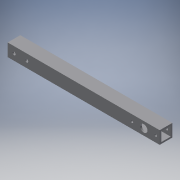
# Autodesk Inventor part: 1x1x12
Saved by Autodesk Inventor 2016 (Build 200138000, 138)
## iProperties
Created: 2016-01-17
Part Number: 1x1x12
Material: Aluminum 6061
Document SubType Name: Modeling
Designer: gus
Density: 2.7 g/cm^3
Appearance: Aluminum - Flat
Mass: 227.61 g
Surface Area: 544.154 cm^2
Volume: 84.2999 cm^3
User Status: complete
Author: gus
Autodesk Inventor part; units mm, degrees
ref_plane "YZ Plane" through (0, 0, 0) normal (1, 0, 0) x (0, 1, 0)
ref_plane "XZ Plane" through (0, 0, 0) normal (0, 1, 0) x (-1, 0, 0)
ref_plane "XY Plane" through (0, 0, 0) normal (0, 0, 1) x (1, 0, 0)
sketch "Sketch1" plane through (0, 0, 0) normal (1, 0, 0) x (0, 1, 0)
  line L0 (0, 0) -> (25.4, 0)
  line L1 (25.4, 0) -> (25.4, -25.4)
  line L2 (25.4, -25.4) -> (0, -25.4)
  line L3 (0, -25.4) -> (0, 0)
  line L4 (22.225, -3.175) -> (3.175, -3.175)
  line L5 (3.175, -3.175) -> (3.175, -22.225)
  line L6 (3.175, -22.225) -> (22.225, -22.225)
  line L7 (22.225, -22.225) -> (22.225, -3.175)
  dimension "d0" = 25.4
  dimension "d1" = 25.4
  dimension "d2" = 3.175
  constraints: 16 end point, 4 parallel, 2 perpendicular, 1 horizontal, 3 other
  measures "d0" distance of L1.end L2.end
  measures "d1" distance of L0.end L1.end
  measures "d2" distance between parallel lines of L0 L4
extrude "Extrusion1" add sketch "Sketch1" along normal blind 304.8
sketch "Sketch2" plane through (0, 0, 0) normal (0, 0, 1) x (1, 0, 0)
  circle A0 centre (273.05, 12.7) radius 23.8125 construction
  line L0 (0, 25.4) -> (304.8, 25.4) construction
  line L1 (304.8, 25.4) -> (304.8, 0) construction
  circle A1 centre (296.8625, 12.7) radius 2.54
  circle A2 centre (249.2375, 12.7) radius 2.54
  line L2 (304.8, 12.7) -> (0, 12.7) construction
  line L3 (0, 0) -> (0, 25.4) construction
  line L4 (276.7162, 19.05) -> (280.3823, 12.7) construction
  line L5 (280.3823, 12.7) -> (276.7162, 6.35) construction
  line L6 (276.7162, 6.35) -> (269.3838, 6.35) construction
  line L7 (269.3838, 6.35) -> (265.7177, 12.7) construction
  line L8 (265.7177, 12.7) -> (269.3838, 19.05) construction
  line L9 (269.3838, 19.05) -> (276.7162, 19.05) construction
  circle A3 centre (273.05, 12.7) radius 7.3323
  circle A4 centre (12.7, 12.7) radius 3.175
  circle A5 centre (38.1, 12.7) radius 3.175
  dimension "d5" = 47.625
  dimension "d6" = 12.7
  dimension "d7" = 31.75
  dimension "d8" = 5.08
  dimension "d9" = 5.08
  dimension "d10" = 12.7
  dimension "d13" = 6.35
  dimension "d14" = 6.35
  dimension "d15" = 12.7
  dimension "d16" = 25.4
  constraints: 14 end point, 5 centre point, 4 point on line, 2 coincident, 2 midpoint, 2 point on circle, 1 horizontal, 16 other
  measures "d5" diameter of A0
  measures "d6" distance from line of L0 A0.centre
  measures "d7" distance from line of L1 A0.centre
  measures "d8" diameter of A1
  measures "d9" diameter of A2
  measures "d10" distance between parallel lines of L6 L9
  measures "d13" diameter of A4
  measures "d14" diameter of A5
  measures "d15" distance from line of L3 A4.centre
  measures "d16" distance of A4.centre A5.centre
extrude "Extrusion2" cut sketch "Sketch2" against normal blind 25.4
body "Solid1"
